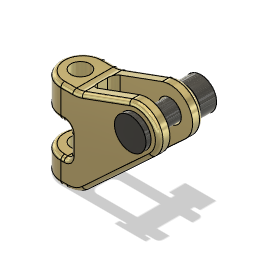
0.885.2490 - Pièce mobile pied de console (Autodesk Fusion 360 design; units mm, degrees)
Autodesk Fusion 360 part; units mm, degrees
note: some values were not read from the file. Set by a fixed rule: which sketch regions a step uses.
sketch "Sketch1" plane through (0, 0, 0) normal (0, 0, 1) x (1, 0, 0)
  line L0 (0, 0) -> (0, 70) construction
  line L1 (0, 0) -> (15.5, 0)
  line L2 (15.5, 0) -> (22.6678, 0)
  line L3 (0, 70) -> (15.5, 70)
  line L4 (15.5, 70) -> (77.5, 70) construction
  line L5 (77.5, 70) -> (77.5, 68) construction
  circle A0 centre (77.5, 68) radius 9
  line L6 (15.5, 70) -> (26.9626, 70)
  line L7 (33.8228, 71.2133) -> (71.3259, 84.908)
  arc A1 (26.9626, 70) -> (33.8228, 71.2133) centre (26.9626, 90) ccw
  line L8 (36.2493, 5.3186) -> (89.7234, 54.7868)
  arc A2 (89.7234, 54.7868) -> (71.3259, 84.908) centre (77.5, 68) ccw
  arc A3 (22.6678, 0) -> (36.2493, 5.3186) centre (22.6678, 20) ccw
  line L9 (77.5, 70) -> (77.5, -60) construction
  line L10 (25, 70) -> (25, 25) construction
  line L11 (0, 0) -> (0, 20)
  line L12 (0, 70) -> (0, 45)
  line L13 (0, 45) -> (20, 45)
  line L14 (0, 20) -> (20, 20)
  line L15 (25, 20) -> (25, 40)
  arc A4 (25, 40) -> (20, 45) centre (20, 40) ccw
  arc A5 (20, 20) -> (25, 25) centre (20, 25) ccw
  point P0 (30.5, 0)
  point P1 (30.5, 70)
  dimension "d1" = 70
  dimension "d2" = 15.5
  dimension "d3" = 15
  dimension "d4" = 15.5
  dimension "d5" = 62
  dimension "d6" = 2
  dimension "d7" = 18
  dimension "d8" = 36
  dimension "d9" = 15
  dimension "d10" = 20
  dimension "d11" = 20
  dimension "d13" = 20
  dimension "d14" = 25
  dimension "d24" = 5
  dimension "d25" = 5
  constraint coincident L0.start L1.start
  constraint coincident L5.end A0.centre
  constraint concentric A0 A2
  constraint tangent L7 A2
  constraint coincident P1 L7
  constraint coincident P1 L6
  constraint tangent L7 A1
  constraint tangent L6 A1
  constraint tangent L8 A2
  constraint coincident P0 L2
  constraint coincident P0 L8
  constraint tangent L2 A3
  constraint tangent L8 A3
  constraint perpendicular L4 L9
  constraint perpendicular L10 L13
  constraint coincident L10 L15.start
  constraint perpendicular L10 L14
  constraint tangent L13 A4
  constraint tangent L15 A4
  constraint parallel L9 L10
  constraint tangent L14 A5
  constraint tangent L10 A5
  measures "d1" distance of L0.start L0.end
  measures "d2" distance of L0.start L1.end
  measures "d3" distance of L1.end P0
  measures "d4" distance of L0.end L3.end
  measures "d5" distance of L3.end L4.end
  measures "d6" distance of L4.end L5.end
  measures "d7" diameter of A0
  measures "d8" diameter of A2
  measures "d9" distance of L3.end P1
  measures "d10" radius of A1
  measures "d11" radius of A3
  measures "d13" distance of L0.start L11.end
  measures "d14" distance of L0.end L12.end
  measures "d24" radius of A4
  measures "d25" radius of A5
extrude "Extrude1" add sketch "Sketch1" along normal blind 35 makes body 1
sketch "Sketch2" plane through (0, 0, 0) normal (0, 1, 0) x (1, 0, 0)
  line L0 (0, 0) -> (0, -35) construction
  line L1 (0, -17.5) -> (17.5, -17.5) construction
  line L2 (22.6678, 0) -> (36.2493, 0) construction
  line L3 (36.2493, 0) -> (36.2493, -35) construction
  line L4 (22.6678, -35) -> (36.2493, -35) construction
  line L5 (22.6678, -35) -> (22.6678, 0) construction
  line L6 (36.2493, 0) -> (89.7234, 0) construction
  line L7 (89.7234, 0) -> (89.7234, -35) construction
  line L8 (89.7234, -35) -> (36.2493, -35) construction
  line L9 (36.2493, -35) -> (36.2493, 0) construction
  line L10 (71.3259, 0) -> (95.5, 0) construction
  line L11 (71.3259, 0) -> (71.3259, -35) construction
  line L12 (71.3259, -35) -> (95.5, -35) construction
  line L13 (89.7234, -35) -> (89.7234, 0) construction
  line L14 (17.5, -35) -> (95.5, -35)
  line L15 (17.5, 0) -> (95.5, 0)
  line L16 (95.5, 0) -> (95.5, -8.5)
  line L17 (95.5, -35) -> (95.5, -26.5)
  arc A0 (17.5, 0) -> (17.5, -35) centre (17.5, -17.5) ccw
  line L18 (86.5, -35) -> (68.5, -35)
  line L19 (86.5, 0) -> (68.5, 0)
  line L20 (68.5, -35) -> (86.5, 0) construction
  line L21 (86.5, -35) -> (68.5, 0) construction
  line L22 (77.5, -17.5) -> (33, -17.5) construction
  line L23 (95.5, -26.5) -> (38, -26.5)
  line L24 (95.5, -8.5) -> (38, -8.5)
  line L25 (33, -17.5) -> (33, -13.5)
  line L26 (33, -17.5) -> (33, -21.5)
  arc A1 (33, -21.5) -> (38, -26.5) centre (38, -21.5) ccw
  arc A2 (38, -8.5) -> (33, -13.5) centre (38, -13.5) ccw
  line L27 (95.5, -8.5) -> (95.5, -26.5)
  line L28 (22.6678, 0) -> (0, 0)
  line L29 (0, 0) -> (0, -35)
  line L30 (22.6678, -35) -> (0, -35)
  point P0 (0, -35)
  dimension "d17" = 17.5
  dimension "d18" = 8.5
  dimension "d19" = 8.5
  dimension "d20" = 44.5
  dimension "d21" = 5
  dimension "d22" = 5
  constraint midpoint L0 L1.start
  constraint coincident L1.end A0.centre
  constraint coincident L1.start A0
  constraint tangent L0 A0
  constraint coincident L12.end L14.end
  constraint tangent L14 A0
  constraint coincident L10.end L15.end
  constraint tangent L15 A0
  constraint coincident L18.end L20.start
  constraint coincident L19.start L20.end
  constraint coincident L18.start L21.start
  constraint coincident L19.end L21.end
  constraint midpoint L21 L22.start
  constraint perpendicular L17 L23
  constraint perpendicular L3 L24
  constraint perpendicular L22 L25
  constraint perpendicular L22 L26
  constraint tangent L26 A1
  constraint tangent L23 A1
  constraint tangent L24 A2
  constraint tangent L25 A2
  constraint perpendicular L24 L27
  constraint coincident L2.start L5.end
  constraint coincident L0.start L28.end
  constraint coincident P0 L0.end
  constraint coincident L4.start L5.start
  measures "d17" distance of L1.start L1.end
  measures "d18" distance of L10.end L16.end
  measures "d19" distance of L12.end L17.end
  measures "d20" distance of L22.start L22.end
  measures "d22" radius of A2
extrude "Extrude2" cut sketch "Sketch2" along normal through all contours A0 L29 L30 | A0 L28 L29 | L23 L24 L25 L26 A1 A2 L27 bodies 1
sketch "Sketch3" plane through (0, 70, 0) normal (0, 1, 0) x (-1, 0, 0)
  arc A0 (-17.5, 0) -> (-17.5, 35) centre (-17.5, 17.5) ccw
  line L0 (-17.5, 35) -> (-26.9626, 35)
  line L1 (-26.9626, 35) -> (-26.9626, 0)
  line L2 (-26.9626, 0) -> (-17.5, 0)
  line L3 (0, 17.5) -> (-15.5, 17.5) construction
  circle A1 centre (-15.5, 17.5) radius 7.5
  dimension "d26" = 15.5
  dimension "d27" = 15
  constraint midpoint A0 L3.start
  constraint coincident L3.end A1.centre
  measures "d26" distance of L3.start L3.end
  measures "d27" diameter of A1
extrude "Extrude3" cut sketch "Sketch3" against normal through all contours A1 bodies 1
fillet "Fillet1" radius 3 28 edges at (18.75, 45, 0) (0, 45, 17.5) (18.75, 45, 35) (23.5355, 43.5355, 35) (25, 32.5, 35) (23.5355, 21.4645, 35) (18.75, 20, 35) (0, 20, 17.5) (18.75, 20, 0) (23.5355, 21.4645, 0) (25, 32.5, 0) (23.5355, 43.5355, 0) (22.2313, 70, 35) (30.4459, 70.3057, 35) (52.5743, 78.0607, 35) (92.8613, 77.3824, 35) (62.9864, 30.0527, 35) (29.9607, 1.3771, 35) (20.0839, 0, 35) (0, 0, 17.5) (20.0839, 0, 0) (29.9607, 1.3771, 0) (62.9864, 30.0527, 0) (92.8613, 77.3824, 0) (52.5743, 78.0607, 0) (30.4459, 70.3057, 0) (22.2313, 70, 0) (0, 70, 17.5) on bodies 1
sketch "Sketch4" plane through (0, 0, 35) normal (0, 0, 1) x (1, 0, 0)
  circle A0 centre (77.5, 68) radius 9
  line L0 (17.5, 3) -> (22.6678, 3)
  arc A1 (22.6678, 3) -> (34.2121, 7.5209) centre (22.6678, 20) ccw
  line L1 (34.2121, 7.5209) -> (87.6861, 56.989)
  arc A2 (87.6861, 56.989) -> (72.3549, 82.09) centre (77.5, 68) ccw
  line L2 (72.3549, 82.09) -> (34.8518, 68.3953)
  arc A3 (26.9626, 67) -> (34.8518, 68.3953) centre (26.9626, 90) ccw
  line L3 (26.9626, 67) -> (17.5, 67)
  line L4 (17.5, 67) -> (17.5, 48)
  line L5 (17.5, 48) -> (20, 48)
  arc A4 (28, 40) -> (20, 48) centre (20, 40) ccw
  line L6 (28, 40) -> (28, 25)
  arc A5 (20, 17) -> (28, 25) centre (20, 25) ccw
  line L7 (20, 17) -> (17.5, 17)
  line L8 (17.5, 17) -> (17.5, 3)
  circle A6 centre (77.5, 68) radius 9
  circle A7 centre (77.5, 68) radius 8
  dimension "d30" = 16
  constraint concentric A0 A7
  measures "d30" diameter of A7
extrude "Extrude4" add sketch "Sketch4" along normal blind 5 and the other way blind 51 separate body contours A7 makes body 2
sketch "Sketch5" plane through (0, 0, 40) normal (0, 0, 1) x (1, 0, 0)
  circle A0 centre (77.5, 68) radius 8
  circle A1 centre (77.5, 68) radius 8
  circle A2 centre (77.5, 68) radius 8
  circle A3 centre (77.5, 68) radius 8
  circle A4 centre (77.5, 68) radius 12.5
  dimension "d35" = 25
  constraint concentric A1 A4
  measures "d35" diameter of A4
extrude "Extrude5" add sketch "Sketch5" against normal blind 4 bodies 2
sketch "Sketch6" plane through (0, 0, -16) normal (0, 0, -1) x (-1, 0, 0)
  circle A0 centre (-77.5, 68) radius 8
  circle A1 centre (-77.5, 68) radius 8
  circle A2 centre (-77.5, 68) radius 12.5
  dimension "d38" = 25
  constraint concentric A1 A2
  measures "d38" diameter of A2
extrude "Extrude6" add sketch "Sketch6" against normal blind 13 bodies 2
equation "d8 = ( 18 * 2 ) * 1 mm"
named bodies: "Pièce mobile", "Axe goupillé"
